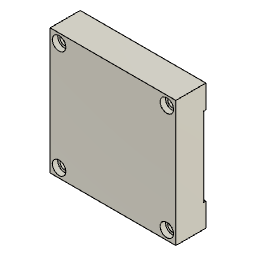
Design 1 GYARB_F_ste (Autodesk Fusion 360 design; units mm, degrees)
Autodesk Fusion 360 part; units mm, degrees
sketch "Sketch1" plane through (0, 0, 0) normal (1, 0, 0) x (0, 1, 0)
  line L0 (10, 35) -> (-10, 35)
  line L1 (-10, 35) -> (-10, -35)
  line L2 (-10, -35) -> (10, -35)
  line L3 (10, 35) -> (-10, -35) construction
  line L4 (-10, 35) -> (10, -35) construction
  line L5 (10, -20) -> (7.5, -20)
  line L6 (7.5, -20) -> (7.5, 20)
  line L7 (7.5, 20) -> (10, 20)
  line L8 (10, -35) -> (10, -20)
  line L9 (10, 20) -> (10, 35)
  dimension "d1" = 20
  dimension "d2" = 70
  dimension "d5" = 2.5
  dimension "d6" = 40
  dimension "d7" = 15
  dimension "d8" = 15
  constraint horizontal L0
  constraint perpendicular L0 L1
  constraint parallel L0 L2
  constraint parallel L1 L8
  constraint coincident L3 origin
  constraint coincident L4 origin
  constraint perpendicular L5 L8
  constraint perpendicular L5 L6
  constraint perpendicular L7 L8
  constraint collinear L8 L9
  measures "d1" distance of L1.end L2.end
  measures "d2" distance of L0.end L1.end
  measures "d5" distance of L6.end L7.end
  measures "d6" distance of L5.end L6.end
  measures "d7" distance of L0.start L7.end
  measures "d8" distance of L2.end L5.start
extrude "Extrude1" add sketch "Sketch1" along normal mid plane 70 makes body 1
sketch "Sketch2" plane through (0, -10, 0) normal (0, -1, 0) x (1, 0, 0)
  line L0 (-35, -35) -> (35, -35)
  line L1 (35, -35) -> (35, 35)
  line L2 (35, 35) -> (-35, 35)
  line L3 (-35, 35) -> (-35, -35)
  circle A0 centre (30, 30) radius 3.75
  circle A1 centre (-30, 30) radius 3.75
  circle A2 centre (-30, -30) radius 3.75
  circle A3 centre (30, -30) radius 3.75
  circle A4 centre (-30, 30) radius 2.5
  circle A5 centre (30, 30) radius 2.5
  circle A6 centre (30, -30) radius 2.5
  circle A7 centre (-30, -30) radius 2.5
  dimension "d13" = 7.5
  dimension "d14" = 7.5
  dimension "d15" = 7.5
  dimension "d16" = 7.5
  dimension "d18" = 5
  dimension "d19" = 5
  dimension "d20" = 5
  dimension "d21" = 5
  constraint concentric A1 A4
  constraint concentric A0 A5
  constraint concentric A3 A6
  constraint concentric A2 A7
  measures "d13" diameter of A0
  measures "d14" diameter of A1
  measures "d15" diameter of A2
  measures "d16" diameter of A3
  measures "d18" diameter of A4
  measures "d19" diameter of A5
  measures "d20" diameter of A6
  measures "d21" diameter of A7
extrude "Extrude2" cut sketch "Sketch2" against normal blind 63 contours A4 | A5 | A6 | A7 bodies 1
extrude "Extrude3" cut sketch "Sketch2" against normal blind 3 contours A0 | A1 | A2 | A3 bodies 1
mirror "Mirror1" about plane through (0, 0, 0) normal (0, 1, 0) of bodies 1 makes body 2
move_body "Move1" bodies 2 to x (1, 0, 0) y (0, 1, 0) z (0, 0, 1) at (0, 35, 0)
delete_body "RemoveBody1" bodies 2
move_body "Move2" bodies 1 to x (1, 0, 0) y (0, 1, 0) z (0, 0, 1) at (0, 4, 0)
sketch "Sketch3" plane through (0, 14, 0) normal (0, 1, 0) x (-1, 0, 0)
  circle A0 centre (-30, 30) radius 2.5
  circle A1 centre (30, 30) radius 2.5
  line L0 (35, 35) -> (-35, 35)
  line L1 (-35, 35) -> (-35, 20)
  line L2 (-35, 20) -> (35, 20)
  line L3 (35, 20) -> (35, 35)
  line L4 (-40, 40) -> (40, 40)
  line L5 (40, 40) -> (40, -40)
  line L6 (40, -40) -> (-40, -40)
  line L7 (-40, -40) -> (-40, 40)
  constraint horizontal L4
  constraint vertical L5
  constraint horizontal L6
  constraint vertical L7
extrude "Extrude4" cut sketch "Sketch3" against normal blind 1.25 contours L0 L1 L2 L3 | L4 L5 L6 L7 bodies 1
sketch "Sketch4" plane through (0, 11.5, 0) normal (0, 1, 0) x (-1, 0, 0)
  line L0 (35, 20) -> (-35, 20)
  line L1 (-35, 20) -> (-35, -20)
  line L2 (-35, -20) -> (35, -20)
  line L3 (35, -20) -> (35, 20)
  line L4 (-38, 22) -> (38, 22)
  line L5 (38, 22) -> (38, -22)
  line L6 (38, -22) -> (-38, -22)
  line L7 (-38, -22) -> (-38, 22)
  line L8 (-38, 22) -> (38, -22) construction
  line L9 (38, 22) -> (-38, -22) construction
  dimension "d11" = 44
  constraint horizontal L4
  constraint perpendicular L4 L5
  constraint parallel L4 L6
  constraint parallel L5 L7
  constraint coincident L8 origin
  constraint coincident L9 origin
  measures "d11" distance of L4.end L5.end
extrude "Extrude5" cut sketch "Sketch4" along normal blind 3 contours L0 L1 L2 L3 | L4 L5 L6 L7 bodies 1
extrude "Extrude6" cut 1 faces at (11.6667, 11.5, 7.3333) along direction (0, -1, 0) blind 2 on bodies 1 bodies 1
extrude "Extrude7" cut 2 faces at (9.4804, 12.75, 24.0151) (9.4804, 12.75, -24.0151) along direction (0, -1, 0) blind 2 on bodies 1 bodies 1
equation "d1 = fäste_bredd"
equation "d2 = fäste_höjd"
equation "d6 = fäste_höjd - 30 mm"
equation "d9 = fäste_extrude"
equation "d13 = skruvfästel"
equation "d14 = skruvfästel"
equation "d15 = skruvfästel"
equation "d16 = skruvfästel"
equation "d18 = skruvhål"
equation "d19 = skruvhål"
equation "d20 = skruvhål"
equation "d21 = skruvhål"
equation "fäste_höjd = 70 mm"
equation "fäste_bredd = 20 mm"
equation "fäste_extrude = 35 mm"
equation "skruvfästel = 7.5 mm"
equation "skruvhål = 5 mm"
